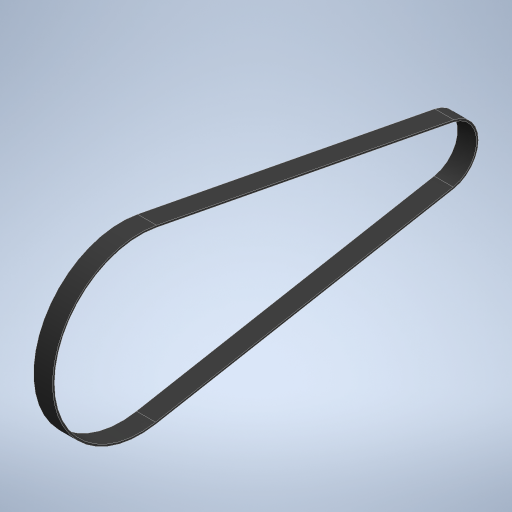
# Autodesk Inventor part: type4
Saved by Autodesk Inventor 2023 (Build 270158000, 158)
## iProperties
Created: 2022-04-24
Part Number: type4
Material: ゴム
Document SubType Name: Modeling
Designer: yuta
Density: 0.93 g/cm^3
Appearance: ゴム - 黒
Author: yuta
Autodesk Inventor part; units mm, degrees
ref_plane "YZ Plane" through (0, 0, 0) normal (1, 0, 0) x (0, 1, 0)
ref_plane "XZ Plane" through (0, 0, 0) normal (0, 1, 0) x (-1, 0, 0)
ref_plane "XY Plane" through (0, 0, 0) normal (0, 0, 1) x (1, 0, 0)
sketch "スケッチ1" plane through (0, 0, 0) normal (1, 0, 0) x (0, 1, 0)
  arc A0 (45.1681, -8.7086) -> (-45.2398, -8.3282) centre (0, 0) ccw
  arc A1 (-16.4172, -164.8953) -> (15.029, -165.0277) centre (-0.6816, -161.9986) ccw
  line L0 (45.1681, -8.7086) -> (15.029, -165.0277)
  line L1 (-45.2398, -8.3282) -> (-16.4172, -164.8953)
  arc A2 (44.1862, -8.5193) -> (-44.2563, -8.1472) centre (0, 0) ccw
  arc A3 (-15.4338, -164.7143) -> (14.0471, -164.8383) centre (-0.6816, -161.9986) ccw
  line L2 (44.1862, -8.5193) -> (14.0471, -164.8383)
  line L3 (-44.2563, -8.1472) -> (-15.4338, -164.7143)
  dimension "d0" = 92
  dimension "d1" = 32
  dimension "d2" = 100
  dimension "d3" = 90
  dimension "d4" = 30
  constraints: 8 end point, 8 point on circle, 8 tangent, 4 centre point, 3 coincident
  measures "d0" diameter of A0
  measures "d1" diameter of A1
  measures "d3" diameter of A2
  measures "d4" diameter of A3
extrude "押し出し1" add sketch "スケッチ1" along normal blind 10
